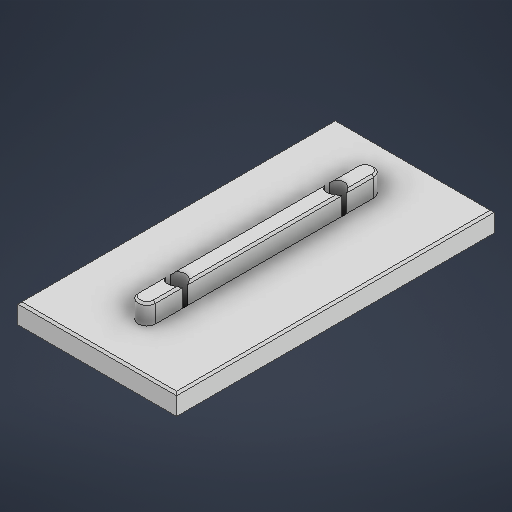
# Autodesk Inventor part: Bolt Slot Covers
Saved by Autodesk Inventor 2026.2 (Build 302298000, 298)
## iProperties
Created: 2026-05-27
Part Number: Bolt Slot Covers
Material: Generic
Document SubType Name: Modeling
Designer: mayhe
Density: 1 g/cm^3
Appearance: Default
Author: mayhe
Autodesk Inventor part; units mm, degrees
ref_plane "YZ Plane" through (0, 0, 0) normal (1, 0, 0) x (0, 1, 0)
ref_plane "XZ Plane" through (0, 0, 0) normal (0, 1, 0) x (-1, 0, 0)
ref_plane "XY Plane" through (0, 0, 0) normal (0, 0, 1) x (1, 0, 0)
sketch "Sketch1" plane through (0, 0, 0) normal (0, 1, 0) x (-1, 0, 0)
  line L0 (20, 40) -> (-20, 40)
  line L1 (-20, 40) -> (-20, -40)
  line L2 (-20, -40) -> (20, -40)
  line L3 (20, -40) -> (20, 40)
  line L4 (20, 40) -> (-20, -40) construction
  line L5 (-20, 40) -> (20, -40) construction
  circle A0 centre (0, 20) radius 2.25
  line L6 (20, 0) -> (36.628, 0)
  circle A1 centre (0, -20) radius 2.25
  point P0 (0, 0)
  dimension "d0" = 40
  dimension "d1" = 80
  dimension "d2" = 4.5
  dimension "d3" = 20
  constraints: 14 end point, 3 midpoint, 2 centre point, 2 horizontal, 2 parallel, 1 perpendicular, 1 symmetric about line, 1 other
  measures "d0" distance of L2.end L1.end
  measures "d1" distance of L1.end L0.end
  measures "d2" diameter of A0
  measures "d3" distance of point (0, 0) A0.centre
extrude "Extrusion1" add sketch "Sketch1" along normal mid plane 5
sketch "Sketch2" plane through (0, 2.5, 0) normal (0, 1, 0) x (1, 0, 0)
  line L0 (0, -27.5) -> (0, 27.5) construction
  arc A0 (-2.175, -27.5) -> (2.175, -27.5) centre (0, -27.5) ccw
  arc A1 (2.175, 27.5) -> (-2.175, 27.5) centre (0, 27.5) ccw
  line L1 (-20, 40) -> (-20, -40) projected
  circle A2 centre (0, 20) radius 2.25 projected
  circle A3 centre (0, -20) radius 2.25 projected
  line L2 (-2.175, -20.5761) -> (-2.175, -27.5)
  line L3 (2.175, -27.5) -> (2.175, -20.5761)
  line L4 (-2.175, 27.5) -> (-2.175, 20.5761)
  line L5 (-2.175, 19.4239) -> (-2.175, -19.4239)
  line L6 (2.175, -19.4239) -> (2.175, 19.4239)
  line L7 (2.175, 20.5761) -> (2.175, 27.5)
  point P0 (0, 0)
  point P1 (0, 0)
  point P2 (-2.175, 0)
  point P3 (-20, 0)
  dimension "d6" = 55
  dimension "d7" = 4.35
  constraints: 16 end point, 12 point on circle, 12 tangent, 9 parallel, 3 midpoint, 2 centre point, 1 horizontal alignment, 1 vertical
  measures "d6" distance of L0.start L0.end
  measures "d7" diameter of A1
extrude "Extrusion2" add sketch "Sketch2" along normal blind 5 contours L2 A3 L3 A0 | L5 A2 L6 A3 | L4 A1 L7 A2
chamfer "Chamfer1" distance 0.5 angle 45 12 edges at (2.175, 7.5, 0) (-2.175, 7.5, 0) (2.175, 7.5, -24.038) (0, 7.5, -29.675) (-2.175, 7.5, -24.038) (0, 7.5, 29.675) (2.175, 7.5, 24.038) (-2.175, 7.5, 24.038) (20, 2.5, 0) (0, 2.5, -40) (-20, 2.5, 0) (0, 2.5, 40)
body "Solid1"
